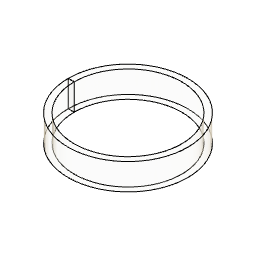
source wall v1 (Autodesk Fusion 360 archive; units mm, degrees)
design "source wall" references "Global Parameters", "source baseplate sketch"
Autodesk Fusion 360 part; units mm, degrees
derive "Derived from Global Parameters v5" from "Global Parameters v5"
derive "Sketch1" from "source baseplate sketch v14"
sketch "Sketch1" plane through (0, 0, 0) normal (0, 1, 0) x (1, 0, 0)
  line L0 (-90, 0) -> (90, 0) construction
  line L1 (-100, 0) -> (100, 0) construction
  line L2 (-90, 0) -> (-100, 0)
  line L3 (-100, 0) -> (-100, -44)
  line L4 (-100, -44) -> (-90, -44)
  line L5 (-90, -44) -> (-90, 0)
  dimension "d1" = 10
  dimension "d2" = 44
  constraint horizontal L2
  constraint vertical L3
  constraint horizontal L4
  constraint vertical L5
  constraint coincident L0.start L2.start
  measures "d1" distance of L3 L5
  measures "d2" distance of L1.start L3.end
revolve "Revolve1" add sketch "Sketch1" angle 359.9 about axis through (0, 0, 1.75) along (0, 0, -1)
convert_to_sheet_metal "ConvertToSheetMetal1"
equation "d1 = pmma_thickness_Ref"
equation "pmma_thickness_Ref = 10 mm" comment "The thickness of the Perspex (Poly Methyl Meth Acrylaat) plate"
equation "rotate_motor_Ref = 117 deg"
